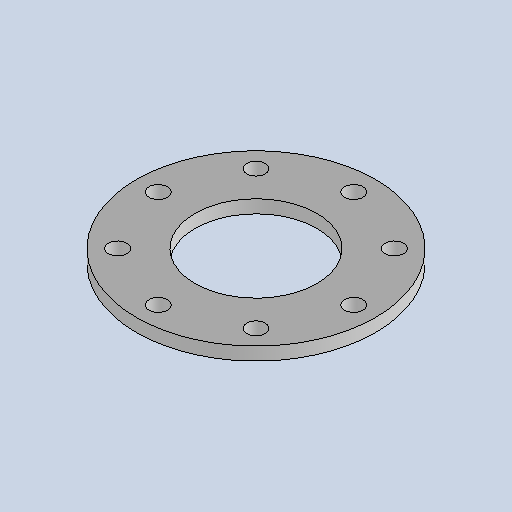
# Autodesk Inventor part: APN 1433 FDS flange DN100
Saved by Autodesk Inventor 2025.3 (Build 293356030, 356C)
## iProperties
Created: 2025-02-13
Part Number: APN 1433 FDS flange DN100
Material: Steel
Document SubType Name: Sheet Metal
Designer: admin
Mass: 2481.74 g
Surface Area: 703.34 cm^2
Volume: 316.145 cm^3
Density: 7.85 g/cm^3
Flat Pattern Width: 22 cm
Flat Pattern Length: 22 cm
Flat Pattern Area: 484 cm^2
Sheet Metal Rule: AISI304 4mm Die 32
Sheet Metal Width: 220,000 mm
Sheet Metal Length: 220,000 mm
Sheet Metal Area: 48400,000 mm^2
Appearance: Default
Author: pokla
Autodesk Inventor part; units mm, degrees
ref_plane "YZ Plane" through (0, 0, 0) normal (1, 0, 0) x (0, 1, 0)
ref_plane "XZ Plane" through (0, 0, 0) normal (0, 1, 0) x (-1, 0, 0)
ref_plane "XY Plane" through (0, 0, 0) normal (0, 0, 1) x (1, 0, 0)
sketch "Sketch2" plane through (0, 0, 0) normal (0, 0, 1) x (1, 0, 0)
  circle A0 centre (0, 0) radius 56
  circle A1 centre (0, 0) radius 110
  dimension "d25" = 112
  dimension "d27" = 220
  measures "d25" diameter of A0
  measures "d27" diameter of A1
extrude "Plate2" add sketch "Sketch2" along normal blind 12
sketch "Sketch3" plane through (0, 0, 12) normal (0, 0, 1) x (1, 0, 0)
  circle A0 centre (-90, 0) radius 8.5
  circle A1 centre (0, 0) radius 90 construction
  dimension "d28" = 180
  dimension "d15" = 17
  constraints: 2 horizontal alignment, 1 centre point, 1 coincident, 2 other
  measures "d15" diameter of A0
extrude "Cut1" cut sketch "Sketch3" against normal blind 12
pattern_circular "Circular Pattern1" count 8 over 360 about axis through (0, 0, -10) along (0, 0, 1) of "Cut1"
equation "\"d17\" = Thickness"
equation "\"d14\" = Thickness"
equation "\"BendReliefWidth\" = Thickness"
equation "\"BendReliefDepth\" = 0.5 * Thickness"
equation "\"CornerReliefSize\" = 4 * Thickness"
equation "\"MinimumRemnant\" = 2 * Thickness"
equation "\"TransitionRadius\" = BendRadius"
equation "\"JacobiRadiusSize\" = BendRadius"
equation "\"GapSize\" = Thickness"
equation "\"Thickness\" = 12"
equation "\"BendRadius\" = 6"
body "Solid3"
